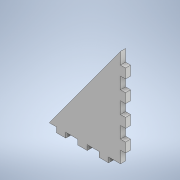
# Autodesk Inventor part: mdf_support
Saved by Autodesk Inventor 2021.2 (Build 252289000, 289)
## iProperties
Created: 2021-03-25
Part Number: mdf_support
Material: Generic
Document SubType Name: Modeling
Designer: yxion
Density: 1 g/cm^3
Appearance: Default
Author: yxion
Autodesk Inventor part; units mm, degrees
ref_plane "YZ Plane" through (0, 0, 0) normal (1, 0, 0) x (0, 1, 0)
ref_plane "XZ Plane" through (0, 0, 0) normal (0, 1, 0) x (-1, 0, 0)
ref_plane "XY Plane" through (0, 0, 0) normal (0, 0, 1) x (1, 0, 0)
sketch "Sketch1" plane through (0, 0, 0) normal (0, 0, 1) x (1, 0, 0)
  line L0 (-51.6543, 109.7487) -> (38.1457, 109.7487) construction
  line L1 (38.1457, -13.2513) -> (-51.6543, -13.2513) construction
  line L2 (-51.6543, -13.2513) -> (-51.6543, 109.7487) construction
  line L3 (38.1457, 94.7487) -> (44.5457, 94.7487)
  line L4 (44.5457, 94.7487) -> (44.5457, 82.7487)
  line L5 (44.5457, 82.7487) -> (38.1457, 82.7487)
  line L6 (38.1457, 82.7487) -> (38.1457, 94.7487)
  line L7 (44.5457, 67.7487) -> (44.5457, 55.7487)
  line L8 (44.5457, 55.7487) -> (38.1457, 55.7487)
  line L9 (38.1457, 55.7487) -> (38.1457, 67.7487)
  line L10 (38.1457, 67.7487) -> (44.5457, 67.7487)
  line L11 (44.5457, 40.7487) -> (44.5457, 28.7487)
  line L12 (44.5457, 28.7487) -> (38.1457, 28.7487)
  line L13 (38.1457, 28.7487) -> (38.1457, 40.7487)
  line L14 (38.1457, 40.7487) -> (44.5457, 40.7487)
  line L15 (44.5457, 13.7487) -> (44.5457, 1.7487)
  line L16 (44.5457, 1.7487) -> (38.1457, 1.7487)
  line L17 (38.1457, 1.7487) -> (38.1457, 13.7487)
  line L18 (38.1457, 13.7487) -> (44.5457, 13.7487)
  line L19 (38.1457, 109.7487) -> (38.1457, -13.2513)
  line L20 (38.1457, -13.2513) -> (-51.6543, -13.2513)
  line L21 (11.1457, -13.2513) -> (23.1457, -13.2513)
  line L22 (23.1457, -13.2513) -> (23.1457, -19.6513)
  line L23 (23.1457, -19.6513) -> (11.1457, -19.6513)
  line L24 (11.1457, -19.6513) -> (11.1457, -13.2513)
  line L25 (-15.8543, -19.6513) -> (-15.8543, -13.2513)
  line L26 (-3.8543, -19.6513) -> (-15.8543, -19.6513)
  line L27 (-3.8543, -13.2513) -> (-3.8543, -19.6513)
  line L28 (-42.8543, -19.6513) -> (-42.8543, -13.2513)
  line L29 (-30.8543, -19.6513) -> (-42.8543, -19.6513)
  line L30 (-30.8543, -13.2513) -> (-30.8543, -19.6513)
  line L31 (-51.6543, -13.2513) -> (38.1457, 109.7487)
  point P0 (0, 0)
  dimension "d0" = 89.8
  dimension "d1" = 123
  dimension "d2" = 12
  dimension "d3" = 6.4
  dimension "d4" = 15
  dimension "d7" = 27
  dimension "d12" = 12
  dimension "d13" = 6.4
  dimension "d14" = 15
  dimension "d17" = 27
  constraints: 64 end point, 6 equal length, 4 horizontal, 2 perpendicular, 2 vertical, 1 collinear, 1 point on line, 37 other
  measures "d0" distance of L1.start L1.end
  measures "d1" distance of L0.end L1.start
  measures "d2" distance of L3.end L4.end
  measures "d3" distance of L3.start L3.end
  measures "d4" distance between parallel lines of L0 L3
  measures "d7" distance of L3.end L7.start
  measures "d12" distance between parallel lines of L22 L24
  measures "d13" distance between parallel lines of L23 L1
  measures "d14" distance from line of L1.start L22
  measures "d17" distance of L23.end L25.start
extrude "Extrusion1" add sketch "Sketch1" along normal blind 6.4
body "Solid1"
